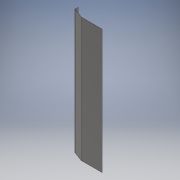
# Autodesk Inventor part: Cover Lower Front
Saved by Autodesk Inventor 2018 (Build 220112000, 112)
## iProperties
Created: 2018-08-07
Part Number: Cover Lower Front
Material: Steel
Document SubType Name: Modeling
Designer: P301319
Density: 7.85 g/cm^3
Appearance: Stainless - Brushed
Author: P301319
Autodesk Inventor part; units mm, degrees
ref_plane "YZ Plane" through (0, 0, 0) normal (1, 0, 0) x (0, 1, 0)
ref_plane "XZ Plane" through (0, 0, 0) normal (0, 1, 0) x (-1, 0, 0)
ref_plane "XY Plane" through (0, 0, 0) normal (0, 0, 1) x (1, 0, 0)
sketch "Sketch1" plane through (0, 0, 0) normal (0, 0, 1) x (1, 0, 0)
  line L0 (0, 0) -> (200, 0)
  line L1 (0, 0) -> (-100, 36.397)
  line L2 (0, 0) -> (106.4178, 0) construction
  line L3 (-100, 36.397) -> (-100, 66.397)
  line L4 (-98.4, 66.397) -> (-98.4, 37.5174)
  line L5 (-98.4, 37.5174) -> (0.2821, 1.6)
  line L6 (0.2821, 1.6) -> (200, 1.6)
  line L7 (-100, 66.397) -> (-98.4, 66.397)
  line L8 (200, 1.6) -> (200, 0)
  dimension "d0" = 200
  dimension "d1" = 160
  dimension "d2" = 100
  dimension "d3" = 30
  dimension "d8" = 1.6
  constraints: 18 end point, 3 horizontal, 2 vertical, 1 equal length, 2 other
  measures "d0" distance of L0.start L0.end
  measures "d1" angle of L2 L1
  measures "d2" horizontal distance of L0.start L1.end
  measures "d3" distance of L1.end L3.end
  measures "d8" distance between parallel lines of L1 L5
extrude "Extrusion1" add sketch "Sketch1" along normal blind 1200
body "Solid1"
